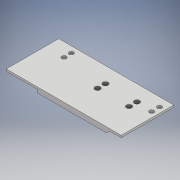
# Autodesk Inventor part: Ball screw right hand support
Saved by Autodesk Inventor 2018 (Build 220112000, 112)
## iProperties
Created: 2017-06-13
Part Number: Ball screw right hand support
Material: Generic
Document SubType Name: Sheet Metal
Designer: m228540
Density: 1 g/cm^3
Appearance: Default
Sheet Metal Rule: Default
Author: m228540
Autodesk Inventor part; units mm, degrees
ref_plane "YZ Plane" through (0, 0, 0) normal (1, 0, 0) x (0, 1, 0)
ref_plane "XZ Plane" through (0, 0, 0) normal (0, 1, 0) x (-1, 0, 0)
ref_plane "XY Plane" through (0, 0, 0) normal (0, 0, 1) x (1, 0, 0)
sketch "Sketch1" plane through (0, 0, 0) normal (0, 0, 1) x (1, 0, 0)
  line L0 (109.5, -50) -> (-109.5, -50)
  line L1 (-109.5, -50) -> (-109.5, 50)
  line L2 (-109.5, 50) -> (109.5, 50)
  line L3 (109.5, 50) -> (109.5, -50)
  constraints: 8 end point, 2 parallel, 1 horizontal, 1 perpendicular
extrude "Extrusion1" add sketch "Sketch1" along normal blind 10
sketch "Sketch6" plane through (0, 0, 0) normal (0, 0, -1) x (-1, 0, 0)
  line L0 (-109.5, 50) -> (109.5, 50) projected
  line L1 (109.5, -50) -> (-109.5, -50) projected
  line L2 (109.5, -50) -> (49.5, -50)
  line L3 (49.5, -50) -> (49.5, 50)
  line L4 (49.5, 50) -> (109.5, 50)
  line L5 (109.5, 50) -> (109.5, -50)
  line L6 (-109.5, -50) -> (-109.5, 50) projected
  line L7 (-109.5, 50) -> (-87.5, 50)
  line L8 (-87.5, 50) -> (-87.5, -50)
  line L9 (-87.5, -50) -> (-109.5, -50)
  line L10 (-109.5, -50) -> (-109.5, 50)
  point P0 (0, 0)
  dimension "d23" = 60
  dimension "d24" = 100
  dimension "d25" = 22
  dimension "d26" = 100
  constraints: 16 end point, 4 parallel, 2 horizontal, 2 perpendicular
  measures "d23" distance of L3.end L4.end
  measures "d24" distance of L2.end L3.end
  measures "d25" distance of L8.end L9.end
  measures "d26" distance of L7.end L8.end
extrude "Extrusion6" cut sketch "Sketch6" against normal blind 6 contours L0 L8 L1 L6 | L0 L5 L1 L3
chamfer "Chamfer1" distance 6 angle 45 1 edges at (87.5, 0, 0)
sketch "Sketch7" plane through (0, 0, 10) normal (0, 0, 1) x (1, 0, 0)
  line L0 (109.5, -50) -> (109.5, 50) projected
  line L1 (109.5, 50) -> (109.5, 18)
  line L2 (109.5, 18) -> (99.5, 18)
  line L3 (109.5, 50) -> (87.5, 50) projected
  line L4 (99.5, 50) -> (99.5, 33)
  line L5 (-109.5, 50) -> (-109.5, -50) projected
  line L6 (-109.5, 50) -> (-73.5, 50) construction
  line L7 (109.5, 50) -> (-109.5, 50) projected
  line L8 (-109.5, 50) -> (-73.5, 50)
  line L9 (-73.5, 50) -> (-73.5, 38)
  line L10 (-73.5, 38) -> (-73.5, 24)
  line L11 (87.5, 50) -> (87.5, -50) projected
  dimension "d32" = 32
  dimension "d34" = 10
  dimension "d36" = 17
  dimension "d37" = 10
  dimension "d41" = 36
  dimension "d42" = 12
  dimension "d43" = 14
  constraints: 14 end point, 3 point on line, 2 perpendicular, 1 collinear, 1 horizontal, 1 vertical
  measures "d32" distance of L0.end L1.end
  measures "d34" distance of L1.end L2.end
  measures "d36" distance of L4.start L4.end
  measures "d37" distance between parallel lines of L0 L4
  measures "d41" distance of L5.start L6.end
  measures "d42" distance of L6.end L9.end
  measures "d43" distance of L9.end L10.end
hole "Hole1" at (99.5, 33, 10) at (99.5, 18, 10) at (-73.5, 24, 10) at (-73.5, 38, 10) direction (0, 0, -1) diameter 8.5 end through all
sketch "Sketch8" plane through (0, 0, 10) normal (0, 0, 1) x (1, 0, 0)
  line L0 (109.5, -50) -> (109.5, 50) projected
  line L1 (109.5, 50) -> (109.5, 20)
  line L2 (109.5, 20) -> (109.5, 5)
  line L3 (109.5, 5) -> (69.5, 5)
  line L4 (69.5, 5) -> (9.5, 5)
  line L5 (9.5, 5) -> (9.5, 20)
  line L6 (69.5, 5) -> (69.5, 20)
  point P0 (0, 0)
  dimension "d58" = 30
  dimension "d59" = 15
  dimension "d60" = 40
  dimension "d61" = 60
  dimension "d62" = 15
  dimension "d70" = 15
  constraints: 12 end point, 3 point on line, 2 perpendicular, 1 vertical
  measures "d58" distance of L0.end L1.end
  measures "d59" distance of L1.end L2.end
  measures "d60" distance of L2.end L3.end
  measures "d61" distance of L3.end L4.end
  measures "d62" distance of L4.end L5.end
  measures "d70" distance of L3.end L6.end
hole "Hole2" at (9.5, 5, 10) at (9.5, 20, 10) at (69.5, 5, 10) at (69.5, 20, 10) direction (0, 0, -1) diameter 10 end through all
thread "Thread1" size "M10x1.5" class "6H" standard "ISO Metric profile" full length
thread "Thread2" size "M10x1.5" class "6H" standard "ANSI Metric M Profile" full length
thread "Thread3" size "M10x1.5" class "6H" standard "ANSI Metric M Profile" full length
thread "Thread4" size "M10x1.5" class "6H" standard "ANSI Metric M Profile" full length
equation "\"d49\" = Thickness"
equation "\"d68\" = Thickness"
equation "\"BendRadius\" = Thickness"
equation "\"BendReliefWidth\" = Thickness"
equation "\"BendReliefDepth\" = 0.5 * Thickness"
equation "\"CornerReliefSize\" = 4 * Thickness"
equation "\"MinimumRemnant\" = 2 * Thickness"
equation "\"TransitionRadius\" = BendRadius"
equation "\"JacobiRadiusSize\" = Thickness"
equation "\"GapSize\" = Thickness"
equation "\"Thickness\" = 0.5"
body "Solid1"
